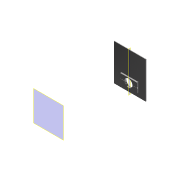
# Autodesk Inventor part: 02_Nanoscopy_Chip
Saved by Autodesk Inventor 2019.4 (Build 234330000, 330)
## iProperties
Created: 2017-12-13
Part Number: 02_Nanoscopy_Chip
Material: Generisch
Document SubType Name: Modeling
Designer: diederichbenedict
Density: 1 g/cm^3
Appearance: Galvanized
Author: diederichbenedict
Autodesk Inventor part; units mm, degrees
ref_plane "YZ Plane" through (0, 0, 0) normal (1, 0, 0) x (0, 1, 0)
ref_plane "XZ Plane" through (0, 0, 0) normal (0, 1, 0) x (-1, 0, 0)
ref_plane "XY Plane" through (0, 0, 0) normal (0, 0, 1) x (1, 0, 0)
sketch "Skizze1" plane through (0, 0, 0) normal (0, 1, 0) x (-1, 0, 0)
  line L0 (0, 0) -> (23.3, 0)
  line L1 (23.3, 0) -> (23.3, 26.8)
  line L2 (23.3, 26.8) -> (0, 26.8)
  line L3 (0, 26.8) -> (0, 0)
  dimension "d0" = 23.3
  dimension "d1" = 26.8
  constraints: 8 end point, 2 parallel, 1 horizontal, 1 perpendicular
  measures "d0" distance of L2.end L1.end
  measures "d1" distance of L1.end L0.end
extrude "Extrusion1" add sketch "Skizze1" along normal blind 0.4
sketch "Skizze2" plane through (0, 0, 0) normal (0, -1, 0) x (1, 0, 0)
  line L0 (0, 0) -> (-23.3, 0) projected
  line L1 (0, 26.8) -> (0, 0) projected
  line L2 (-23.3, 26.8) -> (0, 26.8) projected
  line L3 (-23.3, 0) -> (-23.3, 26.8) projected
  line L4 (-17.8, 3) -> (-5.5, 3)
  line L5 (-5.5, 3) -> (-5.5, 9.8)
  line L6 (-5.5, 9.8) -> (-17.8, 9.8)
  line L7 (-17.8, 9.8) -> (-17.8, 3)
  dimension "d4" = 3
  dimension "d5" = 17
  dimension "d6" = 5.5
  dimension "d7" = 5.5
  constraints: 8 end point, 2 parallel, 1 horizontal, 1 perpendicular
  measures "d4" distance between parallel lines of L4 L0
  measures "d5" distance between parallel lines of L6 L2
  measures "d6" distance between parallel lines of L7 L3
  measures "d7" distance between parallel lines of L1 L5
extrude "Extrusion2" add sketch "Skizze2" along normal blind 1 contours L7 L6 L5 L4
sketch "Skizze3" plane through (0, -1, 0) normal (0, -1, 0) x (1, 0, 0)
  line L0 (-17.8, 3) -> (-5.5, 3) projected
  line L1 (-5.5, 3) -> (-5.5, 9.8) projected
  line L2 (-5.5, 9.8) -> (-17.8, 9.8) projected
  line L3 (-17.8, 9.8) -> (-17.8, 3) projected
  circle A0 centre (-11.65, 6.4) radius 2.9125
  point P0 (0, 0)
  constraints: 1 centre point
extrude "Extrusion3" cut sketch "Skizze3" against normal through all contours A0
ref_plane "Work Plane1" through (-11.65, 0, 0) normal (-1, 0, 0) x (0, 0, 1)
sketch "Sketch5" plane through (0, 0, 26.8) normal (1, 0, 0) x (0, 0, -1)
  line L0 (23.3125, -1) -> (23.3125, 0.4) projected
  line L1 (17.4875, -1) -> (17.4875, 0.4) projected
  circle A0 centre (20.4499, -0.5) radius 0.5025
  point P0 (26.8, 0)
  constraints: 1 centre point
extrude "Extrusion5" cut sketch "Sketch5" against normal through all
ref_plane "Work Plane3" through (-52.1328, -19.1011, -24.6499) normal (0, 1, 0) x (1, 0, 0)
sketch "Sketch6" plane through (-52.1328, -19.1011, -24.6499) normal (0, 1, 0) x (1, 0, 0)
  line L0 (46.6328, -31.0499) -> (52.1328, -31.0499) construction
  line L1 (52.1328, -51.4499) -> (52.1328, -31.0499) construction
  line L2 (28.8328, -51.4499) -> (52.1328, -51.4499) construction
  line L3 (28.8328, -31.0499) -> (28.8328, -51.4499) construction
  line L4 (28.8328, -31.0499) -> (34.3328, -31.0499) construction
  line L5 (34.3328, -31.0499) -> (34.3328, -34.4499) construction
  line L6 (34.3328, -34.4499) -> (46.6328, -34.4499) construction
  line L7 (46.6328, -34.4499) -> (46.6328, -31.0499) construction
  line L8 (6.9828, -36.0499) -> (6.9828, 22.8301) construction
  line L9 (46.6328, -31.5025) -> (34.3328, -31.5025) construction
  line L10 (-16.7355, -31.5025) -> (-33.6581, -41.2728) construction
  line L11 (-33.6581, -41.2728) -> (-33.6581, -21.7322) construction
  line L12 (-33.6581, -21.7322) -> (-16.7355, -31.5025) construction
  point P0 (52.1328, -24.6499)
  point P1 (-28.0172, -31.5025)
  dimension "d16" = 35
  constraints: 6 end point, 1 parallel, 1 point on line, 7 other
  measures "d16" distance from line of point (-28.017, -31.502) L8
hole "Hole1" at (-85.7909, -19.1011, 16.6229) at (-68.8683, -19.1011, 6.8526) at (-85.7909, -19.1011, -2.9177) direction (0, -1, 0) diameter 3.3 depth 12 tip angle 118 counterbore diameter 8 counterbore depth 4
